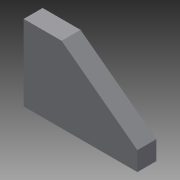
# Autodesk Inventor part: cornerBraceV01
Saved by Autodesk Inventor 2013 (Build 170138000, 138)
## iProperties
Created: 2014-06-26
Part Number: cornerBraceV01
Material: Generic
Document SubType Name: Modeling
Designer: Nano
Density: 1 g/cm^3
Author: Nano
Autodesk Inventor part; units mm, degrees
ref_plane "YZ Plane" through (0, 0, 0) normal (1, 0, 0) x (0, 1, 0)
ref_plane "XZ Plane" through (0, 0, 0) normal (0, 1, 0) x (-1, 0, 0)
ref_plane "XY Plane" through (0, 0, 0) normal (0, 0, 1) x (1, 0, 0)
sketch "Sketch1" plane through (0, 0, 0) normal (0, 0, 1) x (1, 0, 0)
  line L0 (0, 0) -> (38.1, 0)
  line L1 (38.1, 0) -> (38.1, 6.35)
  line L2 (12.7, 25.4) -> (0, 25.4)
  line L3 (0, 25.4) -> (0, 0)
  line L4 (12.7, 25.4) -> (38.1, 6.35)
  dimension "d2" = 6.35
  dimension "d3" = 12.7
  dimension "d4" = 25.4
  dimension "d5" = 38.1
  dimension "d7" = 27.94
  dimension "d8" = 38.1
  constraints: 10 end point, 2 parallel, 1 horizontal, 1 perpendicular
  measures "d2" distance of L1.end L0.end
  measures "d3" distance of L2.start L2.end
  measures "d4" distance of L2.end L0.start
  measures "d5" distance of L0.start L0.end
  measures "d7" distance from line of point (0, 0) L4
  measures "d8" distance from line of point (0, 0) L1
extrude "Extrusion1" add sketch "Sketch1" along normal blind 6.35
body "Solid1"
